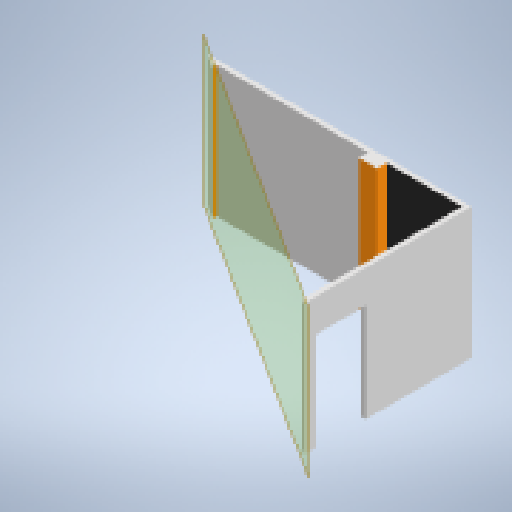
# Autodesk Inventor part: Paredes
Saved by Autodesk Inventor 2024 (Build 280153000, 153)
## iProperties
Created: 2024-04-05
Part Number: Paredes
Material: Genérico
Document SubType Name: Modeling
Designer: sergi
Density: 1 g/cm^3
Appearance: Valor por defecto
Author: sergi
Autodesk Inventor part; units mm, degrees
ref_plane "YZ Plane" through (0, 0, 0) normal (1, 0, 0) x (0, 1, 0)
ref_plane "XZ Plane" through (0, 0, 0) normal (0, 1, 0) x (-1, 0, 0)
ref_plane "XY Plane" through (0, 0, 0) normal (0, 0, 1) x (1, 0, 0)
sketch "Boceto1" plane through (0, 0, 0) normal (0, 1, 0) x (-1, 0, 0)
  line L0 (0, 0) -> (0, -2090)
  line L1 (0, -2090) -> (1560, -2090)
  line L2 (1560, -2090) -> (1560, -1895)
  line L3 (1560, -1895) -> (1935, -1895)
  line L4 (1935, -1895) -> (1935, -2090)
  line L5 (1935, -2090) -> (5065, -2090)
  line L6 (5065, -2090) -> (5065, -1915)
  line L7 (5065, -1915) -> (5250, -1915)
  line L8 (0, 0) -> (0, 310) construction
  line L9 (0, 310) -> (0, 1030) construction
  line L10 (0, 1030) -> (0, 1175)
  line L11 (0, 1175) -> (1645, 1175)
  line L12 (1645, 1175) -> (1645, 1535)
  line L13 (1645, 1535) -> (2010, 1535)
  line L14 (2010, 1535) -> (2010, 1825)
  line L15 (2010, 1825) -> (5120, 1825)
  line L16 (5120, 1825) -> (5120, 1520)
  line L17 (5120, 1520) -> (5300, 1520)
  line L18 (5300, 1520) -> (5250, -1915)
  line L19 (-100, -2190) -> (-100, 0)
  line L20 (-100, 0) -> (-100, 310)
  line L21 (-100, 310) -> (-100, 1030)
  line L22 (-100, 1030) -> (-100, 1275)
  line L23 (-100, 1275) -> (1545, 1275)
  line L24 (1545, 1275) -> (1545, 1635)
  line L25 (1545, 1635) -> (1910, 1635)
  line L26 (1910, 1635) -> (1910, 1925)
  line L27 (1910, 1925) -> (5220, 1925)
  line L28 (5220, 1925) -> (5220, 1620)
  line L29 (5220, 1620) -> (5401.4662, 1620)
  line L30 (5401.4662, 1620) -> (5348.555, -2015)
  line L31 (5348.555, -2015) -> (5165, -2015)
  line L32 (5165, -2015) -> (5165, -2190)
  line L33 (5165, -2190) -> (1835, -2190)
  line L34 (1835, -2190) -> (1835, -1995)
  line L35 (1835, -1995) -> (1660, -1995)
  line L36 (1660, -1995) -> (1660, -2190)
  line L37 (1660, -2190) -> (-100, -2190)
  line L38 (0, 1030) -> (-100, 1030)
  line L39 (0, 0) -> (-100, 0)
  line L40 (1835, -2190) -> (1660, -2190)
  line L41 (5348.555, -2015) -> (5348.555, -2190)
  line L42 (5348.555, -2190) -> (5165, -2190)
  line L43 (5220, 1925) -> (5401.4662, 1925)
  line L44 (5401.4662, 1925) -> (5401.4662, 1620)
  line L45 (1545, 1635) -> (1545, 1925)
  line L46 (1545, 1925) -> (1910, 1925)
  dimension "d0" = 2090
  dimension "d1" = 1560
  dimension "d2" = 195
  dimension "d3" = 375
  dimension "d4" = 195
  dimension "d5" = 3130
  dimension "d6" = 175
  dimension "d8" = 185
  dimension "d10" = 310
  dimension "d11" = 720
  dimension "d12" = 145
  dimension "d13" = 1645
  dimension "d14" = 360
  dimension "d15" = 365
  dimension "d16" = 290
  dimension "d17" = 3110
  dimension "d18" = 305
  dimension "d19" = 180
  dimension "d20" = 100
  constraints: 94 end point, 24 perpendicular, 4 horizontal, 4 point on line, 3 vertical, 1 collinear, 18 other
  measures "d0" distance of L0.start L0.end
  measures "d1" distance of L0.end L1.end
  measures "d2" distance of L1.end L2.end
  measures "d3" distance of L2.end L3.end
  measures "d4" distance of L3.end L4.end
  measures "d5" distance of L4.end L5.end
  measures "d6" distance of L5.end L6.end
  measures "d8" distance of L6.end L7.end
  measures "d10" distance of L0.start L8.end
  measures "d11" distance of L8.end L9.end
  measures "d12" distance of L9.end L10.end
  measures "d13" distance of L10.end L11.end
  measures "d14" distance of L11.end L12.end
  measures "d15" distance of L12.end L13.end
  measures "d16" distance of L13.end L14.end
  measures "d17" distance of L14.end L15.end
  measures "d18" distance of L15.end L16.end
  measures "d19" distance of L16.end L17.end
  measures "d20" distance between parallel lines of L0 L19
extrude "Extrusión1" add sketch "Boceto1" along normal blind 2710 contours L0 L1 L2 L3 L4 L5 L6 L7 L18 L17 L16 L15 L14 L13 L12 L11 L10 L38 L22 L23 L24 L25 L26 L27 L28 L29 L30 L31 L32 L33 L34 L35 L36 L37 L19 L39 | L36 L35 L34 L40 | L32 L31 L41 L42 | L45 L46 L26 L25 | L29 L28 L43 L44
sketch "Boceto2" plane through (0, 0, 0) normal (0, 0, 1) x (1, 0, 0)
  line L0 (0, 0) -> (0, 2030)
  line L1 (0, 0) -> (0, 2710) projected
  line L2 (0, 2030) -> (100, 2030)
  line L3 (100, 0) -> (100, 2710) projected
  line L4 (0, 0) -> (100, 0) projected
  line L5 (100, 0) -> (100, 2710) projected
  line L6 (0, 2710) -> (100, 2710) projected
  line L7 (0, 0) -> (0, 2710) projected
  dimension "d23" = 2030
  constraints: 4 end point, 2 point on line, 1 perpendicular
  measures "d23" distance of L0.start L0.end
extrude "Extrusión2" add sketch "Boceto2" along normal up to surface (1030 mm away) contours L1 L6 L3 L2
sketch "Boceto3" plane through (-5250, 0, -1915) normal (0.9998941, 0, 0.0145545) x (0.0145545, 0, -0.9998941)
  line L0 (-3435.3639, 0) -> (0, 0) projected
  line L1 (0, 0) -> (0, 2710) projected
  line L2 (-3435.3639, 2710) -> (0, 2710) projected
  line L3 (-3435.3639, 0) -> (-3435.3639, 2710) projected
  line L4 (-3435.3639, 0) -> (0, 0) projected
  line L5 (0, 0) -> (-280, 0)
  line L6 (-280, 0) -> (-280, 1120)
  line L7 (-280, 1120) -> (-2610, 1120)
  line L8 (-2610, 1120) -> (-2610, 2470)
  line L9 (-2610, 2470) -> (-280, 2470)
  line L10 (-280, 2470) -> (-280, 1120)
  point P0 (-1838.386, 0)
  dimension "d26" = 280
  dimension "d27" = 1120
  dimension "d28" = 2330
  dimension "d29" = 1350
  constraints: 12 end point, 2 parallel, 2 perpendicular, 1 horizontal, 1 point on line
  measures "d26" distance of L0.end L5.end
  measures "d27" distance of L5.end L6.end
  measures "d28" distance of L8.end L9.end
  measures "d29" distance of L7.end L8.end
extrude "Extrusión3" cut sketch "Boceto3" against normal up to surface (100 mm away) contours L7 L8 L9 L10
ref_plane "Plano division pared" through (-5348.555, 2710, -2190) normal (0.5366261, 0, -0.8438201) x (0.8438201, 0, 0.5366261)
split "Dividir1" plane through (-5348.555, 2710, -2190) removes the side toward (-0.5366261, 0, 0.8438201)
